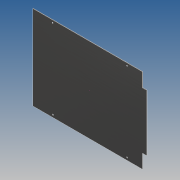
# Autodesk Inventor part: Top_Cover_V1
Saved by Autodesk Inventor 2019 (Build 230136000, 136)
## iProperties
Created: 2020-08-28
Part Number: Top_Cover_V1
Material: Generic
Document SubType Name: Modeling
Designer: voigt
Density: 1 g/cm^3
Appearance: Dark Gray
Author: voigt
Autodesk Inventor part; units mm, degrees
ref_plane "YZ Plane" through (0, 0, 0) normal (1, 0, 0) x (0, 1, 0)
ref_plane "XZ Plane" through (0, 0, 0) normal (0, 1, 0) x (-1, 0, 0)
ref_plane "XY Plane" through (0, 0, 0) normal (0, 0, 1) x (1, 0, 0)
sketch "Sketch1" plane through (0, 0, 0) normal (0, 1, 0) x (-1, 0, 0)
  point P0 (0, 0)
sketch "Sketch2" plane through (0, 0, 0) normal (0, 0, 1) x (1, 0, 0)
  line L0 (0, 297.5) -> (0, -297.5) construction
  line L1 (-402.5, 0) -> (402.5, 0) construction
  line L2 (-287.5, 212.5) -> (287.5, 212.5)
  line L3 (287.5, 212.5) -> (287.5, -212.5)
  line L4 (287.5, -212.5) -> (-287.5, -212.5)
  line L5 (-287.5, -212.5) -> (-287.5, 212.5)
  point P0 (0, 0)
  dimension "d0" = 425
  dimension "d1" = 575
  constraints: 8 end point, 2 parallel, 1 horizontal, 1 perpendicular, 2 other
  measures "d0" distance of L2.end L3.end
  measures "d1" distance of L2.start L2.end
extrude "Extrusion1" add sketch "Sketch2" along normal blind 2
sketch "Sketch3" plane through (0, 0, 2) normal (0, 0, 1) x (1, 0, 0)
  line L0 (287.5, 212.5) -> (-287.5, 212.5) construction
  line L1 (-287.5, 212.5) -> (-287.5, -212.5) construction
  line L2 (-287.5, -212.5) -> (287.5, -212.5) construction
  line L3 (287.5, -212.5) -> (287.5, 212.5) construction
  line L4 (287.5, 212.5) -> (-287.5, 212.5) projected
  line L5 (287.5, 212.5) -> (265.5, 212.5)
  line L6 (265.5, 212.5) -> (265.5, 142.5)
  line L7 (265.5, 142.5) -> (287.5, 142.5)
  line L8 (287.5, 142.5) -> (287.5, 212.5)
  line L9 (287.5, -212.5) -> (265.5, -212.5)
  line L10 (265.5, -212.5) -> (265.5, -142.5)
  line L11 (265.5, -142.5) -> (287.5, -142.5)
  line L12 (287.5, -142.5) -> (287.5, -212.5)
  point P0 (0, 0)
  dimension "d4" = 22
  dimension "d5" = 70
  dimension "d6" = 70
  constraints: 16 end point, 4 parallel, 2 horizontal, 2 perpendicular, 1 point on line
  measures "d4" distance between parallel lines of L3 L6
  measures "d5" distance between parallel lines of L2 L11
  measures "d6" distance between parallel lines of L0 L7
extrude "Extrusion2" cut sketch "Sketch3" against normal blind 2
sketch "Sketch4" plane through (0, 0, 2) normal (0, 0, 1) x (1, 0, 0)
  line L0 (265.5, 142.5) -> (265.5, 212.5) construction
  line L1 (265.5, 212.5) -> (-287.5, 212.5) construction
  line L2 (-287.5, 212.5) -> (-287.5, -212.5) construction
  line L3 (-287.5, -212.5) -> (265.5, -212.5) construction
  line L4 (265.5, -212.5) -> (265.5, -142.5) construction
  line L5 (265.5, -142.5) -> (287.5, -142.5) construction
  line L6 (287.5, -142.5) -> (287.5, 142.5) construction
  line L7 (287.5, 142.5) -> (265.5, 142.5) construction
  line L8 (265.5, 142.5) -> (265.5, 212.5) construction
  line L9 (265.5, 200) -> (-287.5, 200) construction
  line L10 (-287.5, 212.5) -> (265.5, 212.5) construction
  line L11 (-268.0097, 212.5) -> (-268.0097, -212.5) construction
  line L12 (-287.5, -212.5) -> (265.5, -212.5) construction
  line L13 (-287.5, -200) -> (265.5, -200) construction
  point P0 (0, 0)
  point P1 (187.5, 200)
  point P2 (-187.5, 200)
  point P3 (-187.5, -200)
  point P4 (187.5, -200)
  point P5 (-185.9119, -200.0708)
  dimension "d9" = 12.5
  dimension "d10" = 12.5
  dimension "d11" = 100
  dimension "d12" = 100
  dimension "d13" = 100
  dimension "d14" = 100
  constraints: 10 point on line, 6 end point, 3 perpendicular
  measures "d9" distance between parallel lines of L1 L9
  measures "d10" distance between parallel lines of L3 L13
  measures "d11" distance from line of L6 point (187.5, 200)
  measures "d12" distance from line of L6 point (187.5, -200)
  measures "d13" distance from line of L2 point (-187.5, -200)
  measures "d14" distance from line of point (-187.5, 200) L2
hole "Hole1" at (-187.5, 200, 2) at (187.5, 200, 2) at (187.5, -200, 2) at (-185.9119, -200.0708, 2) direction (0, 0, -1) diameter 6 depth 10 tip angle 118
body "Solid1"
